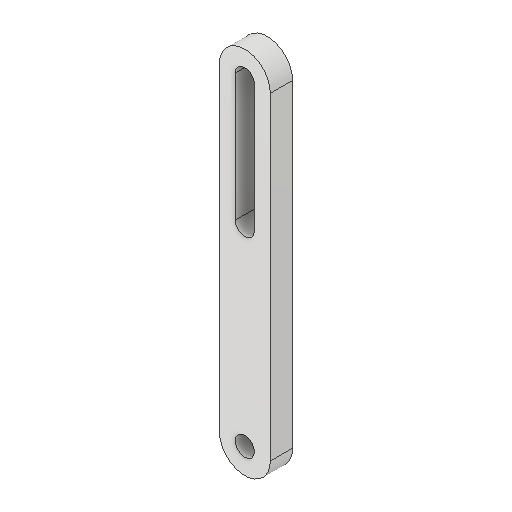
# Autodesk Inventor part: 3DP_PLA_Measurement_Rail_Mounting_Bracket_Long
Saved by Autodesk Inventor 2026.1 (Build 301233000, 233)
## iProperties
Created: 2018-06-16
Part Number: 3DP_PLA_Measurement_Rail_Mounting_Bracket_Long
Material: ABS Plastic
Document SubType Name: Modeling
Designer: Andrzej
Density: 1.06 g/cm^3
Appearance: Smooth - White
Author: Andrzej
Autodesk Inventor part; units mm, degrees
ref_plane "YZ Plane" through (0, 0, 0) normal (1, 0, 0) x (0, 1, 0)
ref_plane "XZ Plane" through (0, 0, 0) normal (0, 1, 0) x (-1, 0, 0)
ref_plane "XY Plane" through (0, 0, 0) normal (0, 0, 1) x (1, 0, 0)
sketch "Sketch1" plane through (0, 0, 0) normal (0, 0, 1) x (1, 0, 0)
  line L0 (0, 25) -> (0, -25) construction
  line L1 (-4, 25) -> (-4, -25)
  line L2 (4, -25) -> (4, 25)
  arc A0 (4, 25) -> (-4, 25) centre (0, 25) ccw
  arc A1 (-4, -25) -> (4, -25) centre (0, -25) ccw
  circle A2 centre (0, -25) radius 1.5
  line L3 (0, 5) -> (0, 25) construction
  line L4 (1.5, 5) -> (1.5, 25)
  line L5 (-1.5, 25) -> (-1.5, 5)
  arc A3 (-1.5, 5) -> (1.5, 5) centre (0, 5) ccw
  arc A4 (1.5, 25) -> (-1.5, 25) centre (0, 25) ccw
  point P0 (0, 0)
  point P1 (0, 15)
  dimension "d0" = 25
  dimension "d1" = 8
  dimension "d2" = 3
  dimension "d3" = 10
  dimension "d4" = 3
  dimension "d5" = 10
  constraints: 16 end point, 8 point on circle, 8 tangent, 5 centre point, 2 midpoint, 2 parallel, 2 point on line, 1 coincident, 1 vertical
  measures "d0" distance of point (0, 0) L0.end
  measures "d1" diameter of A1
  measures "d2" diameter of A2
  measures "d3" distance of point (0, 15) L3.end
  measures "d4" diameter of A4
  measures "d5" distance of L0.start point (0, 15)
extrude "Extrusion1" add sketch "Sketch1" along normal blind 3.5
body "Solid1"
